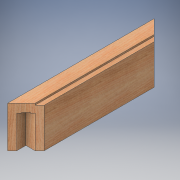
# Autodesk Inventor part: SideWidth
Saved by Autodesk Inventor 2016 (Build 200138000, 138)
## iProperties
Created: 2016-02-09
Part Number: SideWidth
Material: Wood (Birch)
Document SubType Name: Modeling
Designer: ron
Density: 0.55 g/cm^3
Appearance: Birch - Natural Polished
Mass: 4851.38 g
Surface Area: 3661.94 cm^2
Volume: 8820.7 cm^3
Author: ron
Autodesk Inventor part; units mm, degrees
ref_plane "YZ Plane" through (0, 0, 0) normal (1, 0, 0) x (0, 1, 0)
ref_plane "XZ Plane" through (0, 0, 0) normal (0, 1, 0) x (-1, 0, 0)
ref_plane "XY Plane" through (0, 0, 0) normal (0, 0, 1) x (1, 0, 0)
sketch "Sketch1" plane through (0, 0, 0) normal (0, 0, 1) x (1, 0, 0)
  line L0 (0, 0) -> (0, 228.6)
  line L1 (0, 228.6) -> (76.2, 228.6)
  line L2 (76.2, 228.6) -> (76.2, 219.2528)
  line L3 (76.2, 219.2528) -> (101.6, 219.2528)
  line L4 (101.6, 219.2528) -> (101.6, 0)
  line L5 (101.6, 0) -> (0, 0)
  dimension "d0" = 228.6
  dimension "d1" = 76.2
  dimension "d2" = 9.3472
  dimension "d3" = 25.4
  constraints: 12 end point, 5 perpendicular, 1 vertical
  measures "d0" distance of L0.start L0.end
  measures "d1" distance of L0.end L1.end
  measures "d2" distance of L1.end L2.end
  measures "d3" distance of L2.end L3.end
extrude "Extrusion1" add sketch "Sketch1" along normal blind 812.8
sketch "Sketch6" plane through (0, 0, 0) normal (0, -1, 0) x (1, 0, 0)
  line L0 (101.6, 0) -> (101.6, 812.8) projected
  line L1 (0, 812.8) -> (101.6, 711.2) projected
  line L2 (76.2038, 736.5962) -> (25.4038, 736.5962)
  line L3 (25.4038, 736.5962) -> (25.4038, 787.3962)
  line L4 (25.4038, 787.3962) -> (76.2, 736.6)
  point P0 (0, 0)
  point P1 (101.6, 101.6)
  dimension "d31" = 35.9156
  dimension "d32" = 50.8
  dimension "d33" = 50.8
  constraints: 6 end point, 2 point on line, 1 horizontal
  measures "d31" distance of L1.end L2.start
  measures "d32" distance of L2.start L2.end
  measures "d33" distance of L2.end L3.end
extrude "Extrusion4" cut sketch "Sketch6" against normal blind 181.1528
sketch "Sketch7" plane through (25.4038, 0, 736.5962) normal (0, -1, 0) x (1, 0, 0)
  line L0 (76.1962, -634.9962) -> (50.7962, -660.3962)
  line L1 (50.7962, -660.3962) -> (-0.0038, -660.3962)
  line L2 (76.1962, -634.9962) -> (-25.4038, -736.5962) projected
  line L3 (76.1962, -736.5962) -> (76.1962, 76.2038) projected
  line L4 (-0.0038, -660.3962) -> (-0.0038, -711.1962)
  line L5 (-0.0038, -711.1962) -> (50.7962, -660.3962)
  point P0 (76.1962, -25.3962)
  dimension "d39" = 50.8
  dimension "d41" = 90
  dimension "d42" = 50.8
  constraints: 8 end point, 1 collinear, 1 point on line
  measures "d39" distance of L0.end L1.end
  measures "d41" angle of L3 L1
  measures "d42" distance of L1.end L4.end
extrude "Extrusion5" cut sketch "Sketch7" against normal blind 181.1528
chamfer "Chamfer5" distance 101.6 angle 45 1 edges at (101.6, 109.6264, 812.8)
chamfer "Chamfer6" distance 101.6 angle 45 1 edges at (101.6, 109.6264, 0)
sketch "Sketch8" plane through (25.4038, 181.1528, 736.5962) normal (0, -1, 0) x (1, 0, 0)
  line L0 (-25.4038, -736.5962) -> (50.7962, -660.3962) projected
  line L1 (50.7962, -660.3962) -> (38.0981, -673.0942)
  line L2 (38.0981, -673.0942) -> (12.6981, -673.0942)
  line L3 (12.6981, -673.0942) -> (12.6981, -698.4942)
  dimension "d54" = 17.9578
  dimension "d55" = 25.4
  dimension "d56" = 25.4
  constraints: 6 end point, 2 point on line, 1 vertical
  measures "d54" distance of L0.end L1.end
  measures "d55" distance of L1.end L2.end
  measures "d56" distance of L2.end L3.end
extrude "Extrusion6" cut sketch "Sketch8" against normal blind 3.175
sketch "Sketch9" plane through (0, 181.1528, 0) normal (0, -1, 0) x (1, 0, 0)
  line L0 (76.2, 736.6) -> (63.5019, 749.2981)
  line L1 (38.1019, 749.2981) -> (63.5019, 749.2981)
  line L2 (38.1019, 749.2981) -> (38.1019, 774.6981)
  line L3 (38.1019, 774.6981) -> (63.5019, 749.2981)
  line L4 (25.4038, 787.3962) -> (76.2038, 736.5962) projected
  point P0 (0, 0)
  constraints: 8 end point, 1 collinear, 1 perpendicular
extrude "Extrusion8" cut sketch "Sketch9" against normal blind 3.175
body "Solid1"
